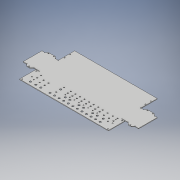
# Autodesk Inventor part: mainCaseFlat
Saved by Autodesk Inventor 2018 (Build 220112000, 112)
## iProperties
Created: 2017-02-09
Part Number: mainCaseFlat
Material: Generic
Document SubType Name: Sheet Metal
Designer: lenord
Density: 1 g/cm^3
Sheet Metal Rule: Default
Appearance: Default
Author: lenord
Autodesk Inventor part; units mm, degrees
ref_plane "YZ Plane" through (0, 0, 0) normal (1, 0, 0) x (0, 1, 0)
ref_plane "XZ Plane" through (0, 0, 0) normal (0, 1, 0) x (-1, 0, 0)
ref_plane "XY Plane" through (0, 0, 0) normal (0, 0, 1) x (1, 0, 0)
sketch "Sketch1" plane through (0, 0, 0) normal (0, 1, 0) x (-1, 0, 0)
  line L0 (257.2308, 49.5858) -> (266.065, 58.42)
  line L1 (266.065, 58.42) -> (283.845, 58.42)
  line L2 (283.845, 58.42) -> (292.6792, 49.5858)
  line L3 (0, 0) -> (0, 139.7) construction
  line L4 (224.155, -55.84) -> (224.155, -142.24)
  line L5 (241.3, 48.26) -> (254.03, 48.26)
  line L6 (295.88, 48.26) -> (313.055, 48.26)
  line L7 (224.155, -53.34) -> (224.155, 139.7) construction
  line L8 (313.055, -53.34) -> (313.055, 48.26)
  line L9 (0, -142.24) -> (0, 139.7) construction
  line L10 (241.3, 48.26) -> (224.155, 48.26)
  line L11 (224.155, 50.8) -> (241.3, 50.8)
  line L12 (241.3, 50.8) -> (241.3, 139.7)
  circle A0 centre (274.955, 54.0029) radius 2.5
  circle A1 centre (253.7883, -59.0829) radius 2.5
  circle A2 centre (283.4217, -59.0829) radius 2.5
  line L13 (274.955, 58.42) -> (274.955, 48.26) construction
  line L14 (226.655, -53.34) -> (237.28, -53.34)
  line L15 (240.4808, -54.6658) -> (249.315, -63.5)
  line L16 (249.315, -63.5) -> (287.895, -63.5)
  line L17 (287.895, -63.5) -> (296.7292, -54.6658)
  line L18 (299.93, -53.34) -> (313.055, -53.34)
  line L19 (241.3, 139.7) -> (0, 139.7)
  line L20 (224.155, -142.24) -> (0, -142.24)
  line L21 (224.155, 50.8) -> (0, 50.8) construction
  circle A3 centre (232.7275, 57.15) radius 2.7432
  circle A4 centre (232.7275, 133.35) radius 2.7432
  line L22 (224.155, 95.25) -> (241.3, 95.25) construction
  line L23 (232.7275, 139.7) -> (232.7275, 50.8) construction
  arc A5 (226.655, -53.34) -> (224.155, -55.84) centre (224.155, -53.34) ccw
  circle A6 centre (218.821, 95.25) radius 2.5
  circle A7 centre (218.821, -112.6067) radius 2.5
  circle A8 centre (218.821, -82.9733) radius 2.5
  arc A9 (240.4808, -54.6658) -> (237.28, -53.34) centre (239.155, -53.34) ccw
  arc A10 (299.93, -53.34) -> (296.7292, -54.6658) centre (298.055, -53.34) ccw
  arc A11 (254.03, 48.26) -> (257.2308, 49.5858) centre (255.905, 48.26) ccw
  arc A12 (292.6792, 49.5858) -> (295.88, 48.26) centre (294.005, 48.26) ccw
  line L24 (-257.2308, 49.5858) -> (-266.065, 58.42)
  line L25 (-266.065, 58.42) -> (-283.845, 58.42)
  line L26 (-283.845, 58.42) -> (-292.6792, 49.5858)
  line L27 (-224.155, -55.84) -> (-224.155, -142.24)
  line L28 (-241.3, 48.26) -> (-254.03, 48.26)
  line L29 (-295.88, 48.26) -> (-313.055, 48.26)
  line L30 (-224.155, -53.34) -> (-224.155, 139.7) construction
  line L31 (-313.055, -53.34) -> (-313.055, 48.26)
  line L32 (-241.3, 48.26) -> (-224.155, 48.26)
  line L33 (-224.155, 50.8) -> (-241.3, 50.8)
  line L34 (-241.3, 50.8) -> (-241.3, 139.7)
  circle A13 centre (-274.955, 54.0029) radius 2.5
  circle A14 centre (-253.7883, -59.0829) radius 2.5
  circle A15 centre (-283.4217, -59.0829) radius 2.5
  line L35 (-274.955, 58.42) -> (-274.955, 48.26) construction
  line L36 (-226.655, -53.34) -> (-237.28, -53.34)
  line L37 (-240.4808, -54.6658) -> (-249.315, -63.5)
  line L38 (-249.315, -63.5) -> (-287.895, -63.5)
  line L39 (-287.895, -63.5) -> (-296.7292, -54.6658)
  line L40 (-299.93, -53.34) -> (-313.055, -53.34)
  line L41 (-241.3, 139.7) -> (0, 139.7)
  line L42 (-224.155, -142.24) -> (0, -142.24)
  line L43 (-224.155, 50.8) -> (0, 50.8) construction
  circle A16 centre (-232.7275, 57.15) radius 2.7432
  circle A17 centre (-232.7275, 133.35) radius 2.7432
  line L44 (-224.155, 95.25) -> (-241.3, 95.25) construction
  line L45 (-232.7275, 139.7) -> (-232.7275, 50.8) construction
  arc A18 (-224.155, -55.84) -> (-226.655, -53.34) centre (-224.155, -53.34) ccw
  circle A19 centre (-218.821, 95.25) radius 2.5
  circle A20 centre (-218.821, -112.6067) radius 2.5
  circle A21 centre (-218.821, -82.9733) radius 2.5
  arc A22 (-237.28, -53.34) -> (-240.4808, -54.6658) centre (-239.155, -53.34) ccw
  arc A23 (-296.7292, -54.6658) -> (-299.93, -53.34) centre (-298.055, -53.34) ccw
  arc A24 (-257.2308, 49.5858) -> (-254.03, 48.26) centre (-255.905, 48.26) ccw
  arc A25 (-295.88, 48.26) -> (-292.6792, 49.5858) centre (-294.005, 48.26) ccw
  circle A26 centre (-198.0051, 229.7957) radius 5
  circle A27 centre (-198.0051, 229.7957) radius 10.75 construction
  line L46 (-206.9953, 246.7597) -> (-189.8978, 246.7597) construction
  line L47 (-189.8978, 246.7597) -> (-189.8978, 242.7114) construction
  line L48 (-189.8978, 242.7114) -> (-206.9953, 242.7114) construction
  line L49 (-206.9953, 242.7114) -> (-206.9953, 246.7597) construction
  circle A28 centre (-179.07, 122.5) radius 5
  circle A29 centre (-179.07, 122.5) radius 10.75 construction
  circle A30 centre (-154.345, 122.5) radius 5
  circle A31 centre (-154.345, 122.5) radius 10.75 construction
  circle A32 centre (-129.62, 122.5) radius 5
  circle A33 centre (-129.62, 122.5) radius 10.75 construction
  circle A34 centre (-104.895, 122.5) radius 5
  circle A35 centre (-104.895, 122.5) radius 10.75 construction
  circle A36 centre (-80.17, 122.5) radius 5
  circle A37 centre (-80.17, 122.5) radius 10.75 construction
  circle A38 centre (-55.445, 122.5) radius 5
  circle A39 centre (-55.445, 122.5) radius 10.75 construction
  circle A40 centre (-30.72, 122.5) radius 5
  circle A41 centre (-30.72, 122.5) radius 10.75 construction
  circle A42 centre (-5.995, 122.5) radius 5
  circle A43 centre (-5.995, 122.5) radius 10.75 construction
  circle A44 centre (18.73, 122.5) radius 5
  circle A45 centre (18.73, 122.5) radius 10.75 construction
  circle A46 centre (43.455, 122.5) radius 5
  circle A47 centre (43.455, 122.5) radius 10.75 construction
  circle A48 centre (68.18, 122.5) radius 5
  circle A49 centre (68.18, 122.5) radius 10.75 construction
  circle A50 centre (92.905, 122.5) radius 5
  circle A51 centre (92.905, 122.5) radius 10.75 construction
  circle A52 centre (-141.9825, 101.4838) radius 5
  circle A53 centre (-141.9825, 101.4838) radius 10.75 construction
  circle A54 centre (-154.9768, 228.869) radius 10.5 construction
  circle A55 centre (-154.9768, 228.869) radius 3.5
  line L50 (-161.7198, 245.7266) -> (-144.4768, 245.7266) construction
  line L51 (-144.4768, 245.7266) -> (-144.4768, 241.5684) construction
  line L52 (-144.4768, 241.5684) -> (-161.7198, 241.5684) construction
  line L53 (-161.7198, 241.5684) -> (-161.7198, 245.7266) construction
  circle A56 centre (-129.62, 75.565) radius 3.5
  circle A57 centre (-129.62, 75.565) radius 10.5 construction
  circle A58 centre (-114.9114, 228.3591) radius 2.5
  line L54 (-118.333, 235.7128) -> (-112.852, 235.7128) construction
  line L55 (-112.852, 235.7128) -> (-112.852, 232.4648) construction
  line L56 (-112.852, 232.4648) -> (-118.333, 232.4648) construction
  line L57 (-118.333, 232.4648) -> (-118.333, 235.7128) construction
  circle A59 centre (-96.09, 228.869) radius 3.25
  circle A60 centre (-96.09, 228.869) radius 6.5 construction
  circle A61 centre (-129.62, 89.215) radius 2.5
  circle A62 centre (-129.62, 59.055) radius 3.25
  circle A63 centre (-129.62, 59.055) radius 6.5 construction
  circle A64 centre (-104.895, 89.215) radius 2.5
  circle A65 centre (-104.895, 75.565) radius 10.5 construction
  circle A66 centre (-104.895, 75.565) radius 3.5
  circle A67 centre (-104.895, 59.055) radius 6.5 construction
  circle A68 centre (-104.895, 59.055) radius 3.25
  circle A69 centre (-80.17, 89.215) radius 2.5
  circle A70 centre (-80.17, 75.565) radius 10.5 construction
  circle A71 centre (-80.17, 75.565) radius 3.5
  circle A72 centre (-80.17, 59.055) radius 6.5 construction
  circle A73 centre (-80.17, 59.055) radius 3.25
  circle A74 centre (-55.445, 89.215) radius 2.5
  circle A75 centre (-55.445, 75.565) radius 10.5 construction
  circle A76 centre (-55.445, 75.565) radius 3.5
  circle A77 centre (-55.445, 59.055) radius 6.5 construction
  circle A78 centre (-55.445, 59.055) radius 3.25
  circle A79 centre (-30.72, 89.215) radius 2.5
  circle A80 centre (-30.72, 75.565) radius 10.5 construction
  circle A81 centre (-30.72, 75.565) radius 3.5
  circle A82 centre (-30.72, 59.055) radius 6.5 construction
  circle A83 centre (-30.72, 59.055) radius 3.25
  circle A84 centre (-5.995, 89.215) radius 2.5
  circle A85 centre (-5.995, 75.565) radius 10.5 construction
  circle A86 centre (-5.995, 75.565) radius 3.5
  circle A87 centre (-5.995, 59.055) radius 6.5 construction
  circle A88 centre (-5.995, 59.055) radius 3.25
  circle A89 centre (18.73, 89.215) radius 2.5
  circle A90 centre (18.73, 75.565) radius 10.5 construction
  circle A91 centre (18.73, 75.565) radius 3.5
  circle A92 centre (18.73, 59.055) radius 6.5 construction
  circle A93 centre (18.73, 59.055) radius 3.25
  circle A94 centre (43.455, 89.215) radius 2.5
  circle A95 centre (43.455, 75.565) radius 10.5 construction
  circle A96 centre (43.455, 75.565) radius 3.5
  circle A97 centre (43.455, 59.055) radius 6.5 construction
  circle A98 centre (43.455, 59.055) radius 3.25
  circle A99 centre (-117.2575, 101.4838) radius 10.75 construction
  circle A100 centre (-117.2575, 101.4838) radius 5
  circle A101 centre (-67.8075, 101.4838) radius 10.75 construction
  circle A102 centre (-67.8075, 101.4838) radius 5
  circle A103 centre (-43.0825, 101.4838) radius 5
  circle A104 centre (-43.0825, 101.4838) radius 10.75 construction
  circle A105 centre (6.3675, 101.4838) radius 10.75 construction
  circle A106 centre (6.3675, 101.4838) radius 5
  circle A107 centre (31.0925, 101.4838) radius 5
  circle A108 centre (31.0925, 101.4838) radius 10.75 construction
  circle A109 centre (-158.0537, 81.7562) radius 3.5
  circle A110 centre (-158.0537, 81.7562) radius 10.5 construction
  circle A111 centre (-158.0537, 61.1188) radius 6.5 construction
  circle A112 centre (-158.0537, 61.1188) radius 3.25
  line L58 (-240.5298, 172.4522) -> (-235.6099, 172.4522) construction
  line L59 (-235.6099, 172.4522) -> (-235.6099, 167.5324) construction
  line L60 (-235.6099, 167.5324) -> (-240.5298, 167.5324) construction
  line L61 (-240.5298, 167.5324) -> (-240.5298, 172.4522) construction
  circle A113 centre (-172.2706, 99.2981) radius 5
  circle A114 centre (-172.2706, 99.2981) radius 10.75 construction
  circle A115 centre (-186.4875, 81.7562) radius 10.5 construction
  circle A116 centre (-186.4875, 81.7562) radius 3.5
  circle A117 centre (-186.4875, 61.1188) radius 6.5 construction
  circle A118 centre (-186.4875, 61.1188) radius 3.25
  circle A119 centre (80.5425, 101.4838) radius 6.5 construction
  circle A120 centre (80.5425, 101.4838) radius 3.25
  circle A121 centre (80.5425, 77.3538) radius 5
  circle A122 centre (80.5425, 77.3538) radius 10.75 construction
  circle A123 centre (80.5425, 59.055) radius 6.5 construction
  circle A124 centre (80.5425, 59.055) radius 3.25
  line L62 (-102.3863, 240.0967) -> (-90.7748, 240.0967) construction
  line L63 (-90.7748, 240.0967) -> (-90.7748, 236.8585) construction
  line L64 (-90.7748, 236.8585) -> (-102.3863, 236.8585) construction
  line L65 (-102.3863, 236.8585) -> (-102.3863, 240.0967) construction
  circle A125 centre (-210.185, 81.7562) radius 3.5
  circle A126 centre (-210.185, 81.7562) radius 10.5 construction
  circle A127 centre (-210.185, 59.055) radius 6.5 construction
  circle A128 centre (-210.185, 59.055) radius 3.25
  circle A129 centre (-210.185, 68.58) radius 2.5
  line L66 (-330.0315, 119.0778) -> (-248.3728, 119.0778) construction
  line L67 (-248.3728, 119.0778) -> (-248.3728, 119.8138) construction
  line L68 (-248.3728, 119.8138) -> (-330.0315, 119.8138) construction
  line L69 (-330.0315, 119.8138) -> (-330.0315, 119.0778) construction
  line L70 (59.1952, 159.9316) -> (63.2213, 159.9316) construction
  line L71 (63.2213, 159.9316) -> (63.2213, 155.9055) construction
  line L72 (63.2213, 155.9055) -> (59.1952, 155.9055) construction
  line L73 (59.1952, 155.9055) -> (59.1952, 159.9316) construction
  circle A130 centre (-197.861, 99.2981) radius 3.25
  circle A131 centre (-197.861, 99.2981) radius 6.5 construction
  line L74 (-202.7888, 31.6249) -> (-199.5308, 31.6249) construction
  line L75 (-199.5308, 31.6249) -> (-199.5308, 28.367) construction
  line L76 (-199.5308, 28.367) -> (-202.7888, 28.367) construction
  line L77 (-202.7888, 28.367) -> (-202.7888, 31.6249) construction
  circle A132 centre (199.39, 122.5) radius 10.75 construction
  circle A133 centre (199.39, 122.5) radius 5
  circle A134 centre (199.39, 85.95) radius 3.5
  circle A135 centre (199.39, 85.95) radius 10.5 construction
  circle A136 centre (199.39, 104.225) radius 2.5
  circle A137 centre (199.39, 64.95) radius 3.25
  circle A138 centre (199.39, 64.95) radius 6.5 construction
  circle A139 centre (170.053, 122.5) radius 5
  circle A140 centre (170.053, 122.5) radius 10.75 construction
  line L78 (193.0383, 161.4795) -> (214.3619, 161.4795) construction
  line L79 (214.3619, 161.4795) -> (214.3619, 143.1563) construction
  line L80 (214.3619, 143.1563) -> (193.0383, 143.1563) construction
  line L81 (193.0383, 143.1563) -> (193.0383, 161.4795) construction
  line L82 (164.7951, 158.772) -> (183.7945, 158.772) construction
  line L83 (183.7945, 158.772) -> (183.7945, 139.7726) construction
  line L84 (183.7945, 139.7726) -> (164.7951, 139.7726) construction
  line L85 (164.7951, 139.7726) -> (164.7951, 158.772) construction
  circle A141 centre (170.053, 101.4838) radius 6.5 construction
  circle A142 centre (170.053, 101.4838) radius 3.25
  circle A143 centre (170.053, 80.4838) radius 3.5
  circle A144 centre (170.053, 80.4838) radius 10.5 construction
  line L86 (134.8346, 158.5069) -> (158.6119, 158.5069) construction
  line L87 (158.6119, 158.5069) -> (158.6119, 140.3043) construction
  line L88 (158.6119, 140.3043) -> (134.8346, 140.3043) construction
  line L89 (134.8346, 140.3043) -> (134.8346, 158.5069) construction
  circle A145 centre (143.178, 122.5) radius 10.75 construction
  circle A146 centre (143.178, 122.5) radius 5
  circle A147 centre (143.178, 101.4838) radius 3.25
  circle A148 centre (143.178, 101.4838) radius 6.5 construction
  circle A149 centre (143.178, 80.4838) radius 10.5 construction
  circle A150 centre (143.178, 80.4838) radius 3.5
  line L90 (239.155, -53.34) -> (240.4808, -54.6658) construction
  line L91 (298.055, -53.34) -> (296.7292, -54.6658) construction
  line L92 (244.8979, -59.0829) -> (292.3121, -59.0829) construction
  line L93 (-296.7292, -54.6658) -> (-298.055, -53.34) construction
  line L94 (-240.4808, -54.6658) -> (-239.155, -53.34) construction
  line L95 (-292.3121, -59.0829) -> (-244.8979, -59.0829) construction
  line L96 (-294.005, 48.26) -> (-292.735, 49.53) construction
  line L97 (-255.905, 48.26) -> (-257.175, 49.53) construction
  arc A151 (224.155, 50.8) -> (224.155, 48.26) centre (224.155, 49.53) ccw
  line L98 (255.905, 48.26) -> (257.2308, 49.5858) construction
  line L99 (292.6792, 49.5858) -> (294.005, 48.26) construction
  line L100 (261.6479, 54.0029) -> (288.2621, 54.0029) construction
  line L101 (-224.155, 48.26) -> (-224.155, 50.8) construction
  arc A152 (-224.155, 48.26) -> (-224.155, 50.8) centre (-224.155, 49.53) ccw
  line L102 (-288.2621, 54.0029) -> (-261.6479, 54.0029) construction
  point P0 (232.7275, 95.25)
  point P1 (-232.7275, 95.25)
  dimension "d37" = 224.155
  dimension "d38" = 10.16
  dimension "d39" = 19.05
  dimension "d45" = 45
  dimension "d64" = 2.54
  dimension "d66" = 5
  dimension "d69" = 15
  dimension "d70" = 101.6
  dimension "d71" = 88.9
  dimension "d74" = 241.3
  dimension "d77" = 139.7
  dimension "d78" = 5.4864
  dimension "d79" = 76.2
  dimension "d80" = 6.35
  dimension "d81" = 5.334
  dimension "d82" = 5.334
  dimension "d83" = 29.6333
  dimension "d84" = 59.2667
  dimension "d85" = 29.6333
  dimension "d86" = 59.2667
  dimension "d87" = 3.75
  dimension "d88" = 10
  dimension "d89" = 21.5
  dimension "d90" = 62.23
  dimension "d91" = 17.2
  dimension "d94" = 24.725
  dimension "d99" = 99.3175
  dimension "d100" = 21.0162
  dimension "d109" = 21
  dimension "d110" = 7
  dimension "d111" = 5
  dimension "d112" = 13
  dimension "d113" = 6.5
  dimension "d114" = 8.255
  dimension "d115" = 16.51
  dimension "d116" = 13.65
  dimension "d117" = 111.68
  dimension "d120" = 24.725
  dimension "d127" = 24.725
  dimension "d134" = 74.175
  dimension "d139" = 10.3187
  dimension "d140" = 20.6375
  dimension "d141" = 83.2463
  dimension "d144" = 28.4337
  dimension "d149" = 69.0294
  dimension "d150" = 17.5419
  dimension "d151" = 321.8425
  dimension "d152" = 24.13
  dimension "d153" = 9.525
  dimension "d154" = 31.115
  dimension "d155" = 43.439
  dimension "d156" = 18.275
  dimension "d157" = 18.275
  dimension "d158" = 21
  dimension "d159" = 41.91
  dimension "d160" = 17.2
  dimension "d161" = 21
  dimension "d162" = 26.875
  dimension "d163" = 71.247
  dimension "d164" = 88.9
  dimension "d166" = 88.9
  dimension "d169" = 10.16
  dimension "d171" = 135
  dimension "d172" = 135
  constraints: 153 centre point, 118 end point, 66 coincident, 60 equal radius, 35 symmetric about line, 24 point on circle, 24 point on line, 19 midpoint, 15 collinear, 15 vertical alignment, 14 horizontal, 14 horizontal alignment, 13 equal length, 6 perpendicular, 3 vertical, 2 tangent, 1 parallel, 174 other
  measures "d37" distance from line of L4 L3.start
  measures "d38" distance between parallel lines of L6 L1
  measures "d39" distance of point (294.005, 48.26) L6.end
  measures "d45" angle of L2 L6
  measures "d64" distance between parallel lines of L10 L11
  measures "d66" diameter of A0
  measures "d69" distance of point (298.055, -53.34) L8.start
  measures "d70" distance between parallel lines of L6 L18
  measures "d71" distance of L11.end L12.end
  measures "d74" distance between parallel lines of L12 L3
  measures "d77" distance from line of L3.start L19
  measures "d78" diameter of A4
  measures "d79" distance of A4.centre A3.centre
  measures "d80" distance from line of L19 A4.centre
  measures "d81" distance from line of L7 A6.centre
  measures "d82" distance from line of L4 A8.centre
  measures "d83" distance from line of A2.centre L8
  measures "d84" distance from line of L8 A1.centre
  measures "d85" distance from line of L20 A7.centre
  measures "d86" distance from line of A8.centre L20
  measures "d87" diameter of A9
  measures "d88" diameter of A26
  measures "d89" diameter of A27
  measures "d90" distance from line of A28.centre L34
  measures "d91" distance from line of L41 A28.centre
  measures "d94" distance of A28.centre A30.centre
  measures "d99" distance from line of A52.centre L34
  measures "d100" vertical distance of A52.centre A38.centre
  measures "d109" diameter of A54
  measures "d110" diameter of A55
  measures "d111" diameter of A58
  measures "d112" diameter of A60
  measures "d113" diameter of A59
  measures "d114" distance from line of A62.centre L43
  measures "d115" distance of A57.centre A62.centre
  measures "d116" distance of A57.centre A61.centre
  measures "d117" distance from line of A56.centre L34
  measures "d120" distance of A61.centre A64.centre
  measures "d127" distance of A53.centre A99.centre
  measures "d134" distance of A53.centre A101.centre
  measures "d139" distance from line of A111.centre L43
  measures "d140" distance of A109.centre A112.centre
  measures "d141" distance from line of A109.centre L34
  measures "d144" distance of A110.centre A115.centre
  measures "d149" distance from line of A113.centre L34
  measures "d150" vertical distance of A113.centre A115.centre
  measures "d151" distance from line of A119.centre L34
  measures "d152" distance of A121.centre A120.centre
  measures "d153" distance of A129.centre A128.centre
  measures "d154" distance from line of A128.centre L34
  measures "d155" distance from line of A130.centre L34
  measures "d156" distance of A132.centre A136.centre
  measures "d157" distance of A136.centre A134.centre
  measures "d158" distance of A134.centre A137.centre
  measures "d159" distance from line of A132.centre L12
  measures "d160" distance from line of L19 A132.centre
  measures "d161" distance of A143.centre A141.centre
  measures "d162" distance of A140.centre A145.centre
  measures "d163" distance from line of L12 A140.centre
  measures "d164" distance between parallel lines of L14 L20
  measures "d166" distance from line of L8 L7.start
  measures "d169" distance from line of point (298.055, -53.34) L16
  measures "d171" angle of L18 L91
  measures "d172" angle of L90 L14
extrude "Plate2" add sketch "Sketch1" along normal blind 3.048 contours L0 L1 L2 A12 L6 L8 L18 A10 L17 L16 L15 A9 L14 A5 L4 L20 L42 L27 A18 L36 A22 L37 L38 L39 A23 L40 L31 L29 A25 L26 L25 L24 A24 L28 L32 A152 L33 L34 L41 L19 L12 L11 A151 L10 L5 A11
equation "\"d37\" = 0.5 * d36"
equation "\"BendRadius\" = Thickness"
equation "\"BendReliefWidth\" = Thickness"
equation "\"BendReliefDepth\" = 0.5 * Thickness"
equation "\"CornerReliefSize\" = 4 * Thickness"
equation "\"MinimumRemnant\" = 2 * Thickness"
equation "\"TransitionRadius\" = BendRadius"
equation "\"JacobiRadiusSize\" = Thickness"
equation "\"GapSize\" = Thickness"
equation "\"d14\" = BendRadius"
equation "\"d56\" = d55"
equation "\"d36\" = 448.31"
equation "\"Thickness\" = 3.048"
equation "\"d55\" = 88.9"
body "Solid2"
